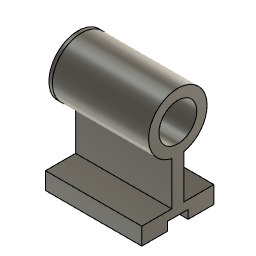
TóthMártonMarcell_1.hazi (Autodesk Fusion 360 design; units mm, degrees)
Autodesk Fusion 360 part; units mm, degrees
note: some values were not read from the file. Set by a fixed rule: which sketch regions a step uses.
sketch "Sketch1" plane through (0, 0, 0) normal (1, 0, 0) x (0, 1, 0)
  line L0 (0, 10) -> (42, 10)
  line L1 (42, 10) -> (42, 0)
  line L2 (42, 0) -> (0, 0)
  line L3 (0, 0) -> (0, 10)
  line L4 (0, 5) -> (42, 5)
  line L5 (15, 0) -> (15, 5)
  line L6 (27, 0) -> (27, 5)
  line L7 (17.5, 52) -> (24.5, 52)
  line L8 (24.5, 52) -> (24.5, 10)
  line L9 (24.5, 10) -> (17.5, 10)
  line L10 (17.5, 10) -> (17.5, 52)
  circle A0 centre (21, 52) radius 17
  circle A1 centre (21, 52) radius 11
  dimension "d1" = 42
  dimension "d2" = 10
  dimension "d4" = 12
  dimension "d5" = 15
  dimension "d6" = 15
  dimension "d7" = 42
  dimension "d8" = 7
  dimension "d9" = 17.5
  dimension "d10" = 34
  dimension "d11" = 22
  constraint horizontal L0
  constraint vertical L1
  constraint horizontal L2
  constraint vertical L3
  constraint coincident L2.end L3.start
  constraint midpoint L3 L4.start
  constraint midpoint L1 L4.end
  constraint coincident L2 L5.start
  constraint coincident L4 L5.end
  constraint perpendicular L4 L5
  constraint coincident L2 L6.start
  constraint coincident L4 L6.end
  constraint perpendicular L4 L6
  constraint horizontal L7
  constraint vertical L8
  constraint horizontal L9
  constraint vertical L10
  constraint coincident L0.start L9
  constraint coincident A0.centre A1.centre
  constraint midpoint L7 A0.centre
  measures "d1" distance of L0.start L0.end
  measures "d2" distance of L0.start L2.end
  measures "d4" distance of L5 L6
  measures "d5" distance of L3 L5
  measures "d6" distance of L1 L6
  measures "d7" distance of L7.end L8.end
  measures "d8" distance of L7.start L7.end
  measures "d9" distance of L1 L8
  measures "d10" diameter of A0
  measures "d11" diameter of A1
extrude "Extrude1" add sketch "Sketch1" along normal blind 56 contours L0 L1 L3 L4 L9 | L0 L8 L9 L10 A0 | L2 L3 L4 L5 | L8 L10 A0 A1 | L8 L10 A0 A1 | L1 L2 L4 L6 makes body 1
extrude "Extrude2" add sketch "Sketch1" against normal blind 2 separate body contours L8 L10 A0 A1 | L8 L10 A0 A1 makes body 2
equation "d9 = ( 35 / 2 ) * 1 mm"
